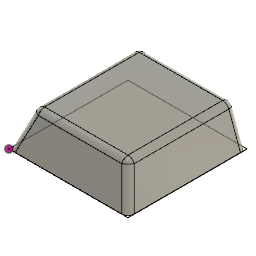
Low Profile Keycap (Autodesk Fusion 360 design; units mm, degrees)
Autodesk Fusion 360 part; units mm, degrees
sketch "Sketch1" plane through (0, 0, 0) normal (0, 0, 1) x (1, 0, 0) in component "Keycap"
  line L0 (0, 0) -> (18, 0)
  line L1 (18, 0) -> (18, 18)
  line L2 (18, 18) -> (0, 18)
  line L3 (0, 18) -> (0, 0)
  dimension "d1" = 18
  dimension "d2" = 18
  constraint horizontal L0
  constraint vertical L1
  constraint horizontal L2
  constraint vertical L3
  constraint coincident L0.start L3.end
  measures "d1" distance of L0.start L0.end
  measures "d2" distance of L0.start L2.end
extrude "Extrude1" add sketch "Sketch1" along normal blind 5.5 in component "Keycap"
draft "Draft1" angle -20 neutral plane through (0, 0, 0) pull (0, 0, -1) 1 faces at (6, 0, 1.8333) in component "Keycap"
draft "Draft2" angle -20 neutral plane through (0, 0, 0) pull (0, 0, -1) 2 faces at (0, 6.6673, 1.8333) (18, 6.6673, 1.8333) in component "Keycap"
fillet "Fillet1" radius 1 4 edges at (1.0009, 1.0009, 2.75) (1.0009, 18, 2.75) (16.9991, 1.0009, 2.75) (16.9991, 18, 2.75) in component "Keycap"
fillet "Fillet1" radius 1 4 edges at (15.9982, 10.0009, 5.5) (9, 18, 5.5) (2.0018, 10.0009, 5.5) (9, 2.0018, 5.5) in component "Keycap"
shell "Shell1" thickness 1 removed faces 1 at (11.6453, 6, 0) in component "Keycap"
sketch "Sketch1 (2)" plane through (0, 0, 4.5) normal (0, 0, -1) x (1, 0, 0)
  line L0 (2.702, -2.702) -> (2.702, -17)
  line L1 (2.702, -17) -> (15.298, -17)
  line L2 (15.298, -17) -> (15.298, -2.702)
  line L3 (15.298, -2.702) -> (2.702, -2.702)
  line L4 (0, -17) -> (0, -0.9397)
  line L5 (0.9397, 0) -> (17.0603, 0)
  line L6 (11.5, -11.4698) -> (6.5, -11.4698)
  line L7 (6.5, -11.4698) -> (6.5, -6.4698)
  line L8 (6.5, -6.4698) -> (11.5, -6.4698)
  line L9 (11.5, -6.4698) -> (11.5, -11.4698)
  line L10 (9, -6.4698) -> (9, 0) construction
  line L11 (6.5, -8.9698) -> (0, -8.9698) construction
  line L12 (11.15, -9.7448) -> (6.85, -9.7448)
  line L13 (6.85, -9.7448) -> (6.85, -8.1948)
  line L14 (6.85, -8.1948) -> (11.15, -8.1948)
  line L15 (11.15, -8.1948) -> (11.15, -9.7448)
  line L16 (9.725, -11.1198) -> (8.275, -11.1198)
  line L17 (8.275, -11.1198) -> (8.275, -6.8198)
  line L18 (8.275, -6.8198) -> (9.725, -6.8198)
  line L19 (9.725, -6.8198) -> (9.725, -11.1198)
  line L20 (8.275, -8.9698) -> (6.5, -8.9698) construction
  line L21 (9, -6.4698) -> (9, -6.8198) construction
  line L22 (11.15, -8.9698) -> (11.5, -8.9698) construction
  line L23 (9, -9.7448) -> (9, -11.4698) construction
  line L24 (8.275, -11.1198) -> (7.925, -11.4698) construction
  line L25 (8.275, -11.1198) -> (8.9157, -11.1198) construction
  line L26 (7.925, -11.4698) -> (6.5, -10.0448)
  line L27 (11.5, -10.0448) -> (10.075, -11.4698)
  line L28 (10.075, -11.4698) -> (9.725, -11.1198) construction
  line L29 (10.075, -6.4698) -> (11.5, -7.8948)
  line L30 (9.725, -6.8198) -> (10.075, -6.4698) construction
  line L31 (8.275, -6.8198) -> (7.925, -6.4698) construction
  line L32 (7.925, -6.4698) -> (6.5, -7.8948)
  dimension "d26" = 5
  dimension "d27" = 5
  dimension "d28" = 1.55
  dimension "d29" = 1.45
  dimension "d30" = 4.3
  dimension "d31" = 4.3
  dimension "d32" = 135
  constraint horizontal L6
  constraint vertical L7
  constraint horizontal L8
  constraint vertical L9
  constraint midpoint L8 L10.start
  constraint midpoint L5 L10.end
  constraint perpendicular L5 L10
  constraint midpoint L7 L11.start
  constraint midpoint L4 L11.end
  constraint perpendicular L4 L11
  constraint horizontal L12
  constraint vertical L13
  constraint horizontal L14
  constraint vertical L15
  constraint horizontal L16
  constraint vertical L17
  constraint horizontal L18
  constraint vertical L19
  constraint midpoint L17 L20.start
  constraint coincident L7 L11.start
  constraint perpendicular L7 L20
  constraint midpoint L18 L21.end
  constraint perpendicular L18 L21
  constraint midpoint L15 L22.start
  constraint coincident L9 L22.end
  constraint perpendicular L9 L22
  constraint midpoint L9 L22.end
  constraint midpoint L12 L23.start
  constraint midpoint L6 L23.end
  constraint perpendicular L12 L23
  constraint horizontal L25
  constraint coincident L6 L24.end
  constraint coincident L7 L26.end
  constraint perpendicular L24 L26
  constraint coincident L9 L27.start
  constraint coincident L6 L27.end
  constraint perpendicular L26 L27
  constraint perpendicular L27 L28
  constraint coincident L8 L29.start
  constraint coincident L9 L29.end
  constraint perpendicular L27 L29
  constraint perpendicular L29 L30
  constraint coincident L8 L31.end
  constraint perpendicular L24 L31
  constraint coincident L7 L32.end
  constraint perpendicular L31 L32
  measures "d26" distance of L6.start L8.end
  measures "d27" distance of L6.start L6.end
  measures "d28" distance of L12.start L14.end
  measures "d29" distance of L16.start L16.end
  measures "d30" distance of L16.start L18.end
  measures "d31" distance of L12.start L12.end
  measures "d32" angle of L24 L25
extrude "Extrude3" add sketch "Sketch1 (2)" along normal blind 4.5 contours L6 L7 L8 L9 L26 L27 L29 L32 in component "Keycap"
component "Keycap" placed x (1, 0, 0) y (0, 1, 0) z (0, 0, 1) at (0, 0, 0)
